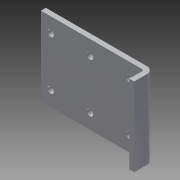
# Autodesk Inventor part: Spacer 3
Saved by Autodesk Inventor 2014 (Build 180170000, 170)
## iProperties
Created: 2014-01-17
Part Number: Spacer 3
Material: Aluminum 6061
Document SubType Name: Sheet Metal
Designer: Michael
Density: 2.71 g/cm^3
Sheet Metal Rule: Default
Appearance: Aluminum - Flat
Author: Michael
Autodesk Inventor part; units mm, degrees
ref_plane "YZ Plane" through (0, 0, 0) normal (1, 0, 0) x (0, 1, 0)
ref_plane "XZ Plane" through (0, 0, 0) normal (0, 1, 0) x (-1, 0, 0)
ref_plane "XY Plane" through (0, 0, 0) normal (0, 0, 1) x (1, 0, 0)
sketch "Sketch1" plane through (0, 0, 0) normal (0, 0, 1) x (1, 0, 0)
  line L0 (0, 0) -> (69.85, 0)
  line L1 (69.85, 0) -> (69.85, 50.8)
  line L2 (69.85, 50.8) -> (0, 50.8)
  line L3 (0, 50.8) -> (0, 0)
  circle A0 centre (6.35, 9.525) radius 2.0701
  circle A1 centre (31.75, 9.525) radius 2.0701
  circle A2 centre (57.15, 9.525) radius 2.0701
  circle A3 centre (6.35, 41.275) radius 2.0701
  circle A4 centre (31.75, 41.275) radius 2.0701
  circle A5 centre (57.15, 41.275) radius 2.0701
  dimension "d4" = 50.8
  dimension "d5" = 69.85
  dimension "d6" = 4.1402
  dimension "d7" = 6.35
  dimension "d8" = 9.525
  dimension "d9" = 25.4
  dimension "d10" = 31.75
  measures "d4" distance of L1.end L0.end
  measures "d5" distance of L0.start L0.end
  measures "d6" diameter of A0
  measures "d7" distance from line of L3 A0.centre
  measures "d8" distance from line of L0 A0.centre
  measures "d9" distance of A0.centre A1.centre
  measures "d10" distance of A0.centre A3.centre
extrude "Plate1" add sketch "Sketch1" along normal blind 3.175
sketch "Sketch2" plane through (66.675, 50.8, 0) normal (1, 0, 0) x (0, 1, 0)
  line L0 (-50.8, 0) -> (0, 0)
  line L1 (0, 0) -> (0, 12.7)
  line L2 (0, 12.7) -> (-50.8, 12.7)
  line L3 (-50.8, 12.7) -> (-50.8, 0)
  constraints: 6 end point, 1 horizontal, 1 perpendicular, 1 vertical
edge flange "Flange1" height 12.7 angle 90 thickness 3.175 bend radius 1.27 thickness toward (1, 0, 0) relief straight relief width 3.175 relief depth 1.5875 edges at (69.85, 25.4, 3.175) wall of the first edge with corners at (66.675, 0, 0) (66.675, 50.8, 0) (66.675, 50.8, 12.7) (66.675, 0, 12.7)
bend "Bend1"
corner "Corner1"
equation "\"d12\" = BendReliefWidth"
equation "\"d13\" = BendReliefDepth"
equation "\"d14\" = MinimumRemnant"
equation "\"d15\" = BendRadius"
equation "\"d19\" = CornerReliefSize"
equation "\"d20\" = GapSize"
equation "\"d21\" = JacobiRadiusSize"
equation "\"BendRadius\" = Thickness"
equation "\"BendReliefWidth\" = Thickness"
equation "\"BendReliefDepth\" = 0.5 * Thickness"
equation "\"CornerReliefSize\" = 4 * Thickness"
equation "\"MinimumRemnant\" = 2 * Thickness"
equation "\"TransitionRadius\" = BendRadius"
equation "\"JacobiRadiusSize\" = BendRadius"
equation "\"GapSize\" = Thickness"
equation "\"d11\" = BendRadius"
equation "\"Thickness\" = 3.175"
body "Solid1"
